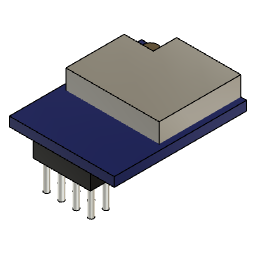
MLH3 v1.0 (Autodesk Fusion 360 archive; units mm, degrees)
design "RA-02"
Autodesk Fusion 360 part; units mm, degrees
sketch "Esquisse1" plane through (0, 0, 0) normal (0, 0, 1) x (1, 0, 0) in component "LoRa RA-02"
  line L0 (0, 0) -> (18, 0)
  line L1 (18, 0) -> (18, -22.7)
  line L2 (18, -22.7) -> (0, -22.7)
  line L3 (0, -22.7) -> (0, 0)
  line L4 (1, 0) -> (17, 0)
  line L5 (17, 0) -> (17, -14)
  line L6 (17, -14) -> (1, -14)
  line L7 (1, -14) -> (1, 0)
  line L8 (13.9, -22.7) -> (4.1, -22.7)
  line L9 (4.1, -22.7) -> (4.1, -17.7)
  line L10 (4.1, -17.7) -> (13.9, -17.7)
  line L11 (13.9, -17.7) -> (13.9, -22.7)
  line L12 (1, 0) -> (6, 0)
  line L13 (6, 0) -> (6, -4)
  line L14 (6, -4) -> (1, -4)
  line L15 (1, -4) -> (1, 0)
  circle A0 centre (3.5142, -2) radius 1.25
  circle A1 centre (5.2, -21.5) radius 0.445
  circle A2 centre (7.74, -21.5) radius 0.445
  circle A3 centre (10.28, -21.5) radius 0.445
  circle A4 centre (12.82, -21.5) radius 0.445
  circle A5 centre (5.2, -18.96) radius 0.445
  circle A6 centre (7.74, -18.96) radius 0.445
  circle A7 centre (10.28, -18.96) radius 0.445
  circle A8 centre (12.82, -18.96) radius 0.445
  dimension "d1" = 18
  dimension "d2" = 22.7
  dimension "d3" = 16
  dimension "d4" = 14
  dimension "d5" = 9.8
  dimension "d6" = 5
  dimension "d7" = 5
  dimension "d8" = 4
  dimension "d9" = 2.5
  dimension "d18" = 0.89
  dimension "d21" = 7.62
  dimension "d22" = 2.54
  dimension "d23" = 1.2
  dimension "d24" = 1.1
  constraint horizontal L0
  constraint vertical L1
  constraint horizontal L2
  constraint vertical L3
  constraint coincident L0.start L3.end
  constraint horizontal L4
  constraint vertical L5
  constraint horizontal L6
  constraint vertical L7
  constraint coincident L0 L4.start
  constraint midpoint L0 L4
  constraint horizontal L8
  constraint vertical L9
  constraint horizontal L10
  constraint vertical L11
  constraint coincident L2 L8.start
  constraint midpoint L2 L8
  constraint horizontal L12
  constraint vertical L13
  constraint horizontal L14
  constraint vertical L15
  measures "d1" distance of L0.start L0.end
  measures "d2" distance of L0.start L2.end
  measures "d3" distance of L4.start L4.end
  measures "d4" distance of L4.start L6.end
  measures "d5" distance of L8.start L8.end
  measures "d6" distance of L8.start L10.end
  measures "d7" distance of L4.start L12.end
  measures "d8" distance of L4.start L14.end
  measures "d9" diameter of A0
  measures "d18" diameter of A1
  measures "d23" distance of L2 A1.centre
  measures "d24" distance of L9 A1.centre
extrude "Extrusion1" add sketch "Esquisse1" along normal blind 1.6 contours L0 L1 L2 L3 L5 L6 L7 L9 L10 L11 L15 | L0 L4 L7 L12 L13 L14 L15 | L0 L4 L5 L6 L7 L13 L14 | L2 L8 L9 L10 L11 | A0 | A1 | A2 | A3 | A4 | A5 | A6 | A7 | A8 makes body 1 in component "LoRa RA-02"
extrude "Extrusion2" add sketch "Esquisse1" against normal blind 2.6 separate body contours L2 L8 L9 L10 L11 | A1 | A2 | A3 | A4 | A5 | A6 | A7 | A8 makes body 2 in component "LoRa RA-02"
extrude "Extrusion3" add sketch "Esquisse1" along normal blind 4.9 separate body contours L0 L4 L5 L6 L7 L13 L14 makes body 3 in component "LoRa RA-02"
extrude "Extrusion4" add sketch "Esquisse1" along normal blind 3 separate body contours A0 makes body 4 in component "LoRa RA-02"
extrude "Extrusion5" add sketch "Esquisse1" against normal blind 5 from surface at -2.6 separate body contours A1 | A2 | A3 | A4 | A5 | A6 | A7 | A8 makes body 5 at (10.077, -19.356, -4.2667) makes body 6 at (8.1712, -21.6098, -5.9333) makes body 7 at (12.617, -21.896, -4.2667) makes body 8 at (8.1712, -19.0698, -5.9333) makes body 9 at (12.617, -19.356, -4.2667) makes body 10 at (5.6312, -21.6098, -5.9333) makes body 11 at (10.077, -21.896, -4.2667) makes body 12 at (5.6312, -19.0698, -5.9333) in component "LoRa RA-02"
component "LoRa RA-02" placed x (1, 0, 0) y (0, 1, 0) z (0, 0, 1) at (0, 0, 0)
named bodies: "PCB", "connecteur", "SX11278", "IPX"

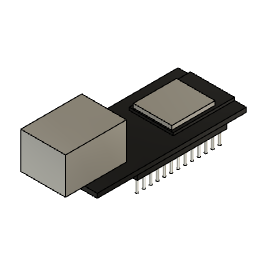
design "WT32-ETH01"
Autodesk Fusion 360 part; units mm, degrees
sketch "Esquisse1" plane through (0, 0, 0) normal (0, 0, 1) x (1, 0, 0) in component "WT32-ETH01"
  line L0 (-12.6, 31.1) -> (12.6, 31.1)
  line L1 (12.6, 31.1) -> (12.6, -23.9)
  line L2 (12.6, -23.9) -> (-12.6, -23.9)
  line L3 (-12.6, -23.9) -> (-12.6, 31.1)
  line L4 (12.6, -9.1479) -> (10.7452, -9.1479)
  line L5 (10.7452, -9.1479) -> (10.7452, 23.8669)
  line L6 (10.7452, 23.8669) -> (12.6, 23.8669)
  line L7 (12.6, 23.8669) -> (12.6, -9.1479)
  line L8 (-12.6, -9.1839) -> (-11, -9.1839)
  line L9 (-11, -9.1839) -> (-11, 24)
  line L10 (-11, 24) -> (-12.6, 24)
  line L11 (-12.6, 24) -> (-12.6, -9.1839)
  circle A0 centre (-11.55, -8) radius 0.445
  circle A1 centre (11.31, -8) radius 0.445
  circle A2 centre (-11.55, -5.46) radius 0.445
  circle A3 centre (11.31, -5.46) radius 0.445
  circle A4 centre (-11.55, -2.92) radius 0.445
  circle A5 centre (11.31, -2.92) radius 0.445
  circle A6 centre (-11.55, -0.38) radius 0.445
  circle A7 centre (11.31, -0.38) radius 0.445
  circle A8 centre (-11.55, 2.16) radius 0.445
  circle A9 centre (11.31, 2.16) radius 0.445
  circle A10 centre (-11.55, 4.7) radius 0.445
  circle A11 centre (11.31, 4.7) radius 0.445
  circle A12 centre (-11.55, 7.24) radius 0.445
  circle A13 centre (11.31, 7.24) radius 0.445
  circle A14 centre (-11.55, 9.78) radius 0.445
  circle A15 centre (11.31, 9.78) radius 0.445
  circle A16 centre (-11.55, 12.32) radius 0.445
  circle A17 centre (11.31, 12.32) radius 0.445
  circle A18 centre (-11.55, 14.86) radius 0.445
  circle A19 centre (11.31, 14.86) radius 0.445
  circle A20 centre (-11.55, 17.4) radius 0.445
  circle A21 centre (11.31, 17.4) radius 0.445
  circle A22 centre (-11.55, 19.94) radius 0.445
  circle A23 centre (11.31, 19.94) radius 0.445
  circle A24 centre (-11.55, 22.48) radius 0.445
  circle A25 centre (11.31, 22.48) radius 0.445
  dimension "d1" = 25.2
  dimension "d2" = 55
  dimension "d13" = 0.89
  dimension "d16" = 22.86
  dimension "d17" = 30.48
  dimension "d18" = 1.05
  constraint horizontal L0
  constraint vertical L1
  constraint horizontal L2
  constraint vertical L3
  constraint horizontal L4
  constraint vertical L5
  constraint horizontal L6
  constraint vertical L7
  constraint coincident L1 L4.start
  constraint horizontal L8
  constraint vertical L9
  constraint horizontal L10
  constraint vertical L11
  constraint coincident L3 L8.start
  measures "d1" distance of L0.start L0.end
  measures "d2" distance of L0.start L2.end
  measures "d13" diameter of A0
  measures "d18" distance of L11 A0.centre
extrude "Extrusion1" add sketch "Esquisse1" along normal blind 1.6 contours L0 L1 L2 L3 L4 L5 L6 L8 L9 L10 | L3 L8 L9 L10 L11 | L1 L4 L5 L6 L7 | A0 | A1 | A2 | A3 | A4 | A5 | A6 | A7 | A8 | A9 | A10 | A11 | A12 | A13 | A14 | A15 | A16 | A17 | A18 | A19 | A20 | A21 | A22 | A23 | A24 | A25 makes body 1 in component "WT32-ETH01"
extrude "Extrusion2" add sketch "Esquisse1" against normal blind 1.7 separate body contours L3 L8 L9 L10 L11 | L1 L4 L5 L6 L7 | A0 | A1 | A2 | A3 | A4 | A5 | A6 | A7 | A8 | A9 | A10 | A11 | A12 | A13 | A14 | A15 | A16 | A17 | A18 | A19 | A20 | A21 | A22 | A23 | A24 | A25 makes body 2 at (11.3634, 12.862, 0) makes body 3 at (-12.6, 1.8774, -0.5667) in component "WT32-ETH01"
sketch "Esquisse2" plane through (0, 0, 1.6) normal (0, 0, 1) x (-1, 0, 0) in component "WT32-ETH01"
  line L0 (12.6, -31.1) -> (12.6, 23.9)
  line L1 (12.6, 23.9) -> (-12.6, 23.9)
  line L2 (-12.6, 23.9) -> (-12.6, -31.1)
  line L3 (-12.6, -31.1) -> (12.6, -31.1)
  line L4 (8, -8.5) -> (-8.2548, -8.5)
  line L5 (-8.2548, -8.5) -> (-8.2548, -31.1)
  line L6 (-8.2548, -31.1) -> (8, -31.1)
  line L7 (8, -31.1) -> (8, -8.5)
  line L8 (8.5, 8.5) -> (-8, 8.5)
  line L9 (-8, 8.5) -> (-8, 31)
  line L10 (-8, 31) -> (8.5, 31)
  line L11 (8.5, 31) -> (8.5, 8.5)
  line L12 (7, -9) -> (-7.213, -9)
  line L13 (-7.213, -9) -> (-7.213, -24.9545)
  line L14 (-7.213, -24.9545) -> (7, -24.9545)
  line L15 (7, -24.9545) -> (7, -9)
  constraint horizontal L4
  constraint vertical L5
  constraint horizontal L6
  constraint vertical L7
  constraint coincident L3 L5.end
  constraint horizontal L8
  constraint vertical L9
  constraint horizontal L10
  constraint vertical L11
  constraint horizontal L12
  constraint vertical L13
  constraint horizontal L14
  constraint vertical L15
extrude "Extrusion3" add sketch "Esquisse2" along normal blind 13.5 separate body contours L1 L8 L9 L11 | L1 L9 L10 L11 makes body 4 in component "WT32-ETH01"
extrude "Extrusion4" add sketch "Esquisse2" along normal blind 1 separate body contours L3 L4 L5 L6 L7 makes body 5 in component "WT32-ETH01"
extrude "Extrusion5" add sketch "Esquisse2" along normal blind 2.5 separate body contours L12 L13 L14 L15 makes body 6 in component "WT32-ETH01"
extrude "Extrusion6" add sketch "Esquisse1" against normal blind 5 from surface at -1.7 separate body contours A0 | A1 | A2 | A3 | A4 | A5 | A6 | A7 | A8 | A9 | A10 | A11 | A12 | A13 | A14 | A15 | A16 | A17 | A18 | A19 | A20 | A21 | A22 | A23 | A24 | A25 makes body 7 at (-11.1056, -2.9422, -5.0333) makes body 8 at (-11.4295, 7.6684, -5.0333) makes body 9 at (-11.753, 17.004, -3.3667) makes body 10 at (11.107, 19.544, -3.3667) makes body 11 at (11.7412, 9.8898, -5.0333) makes body 12 at (11.4305, 0.0484, -5.0333) makes body 13 at (11.4305, -7.5716, -5.0333) makes body 14 at (11.7544, 2.1378, -5.0333) makes body 15 at (11.7412, 12.4298, -5.0333) makes body 16 at (11.107, 22.084, -3.3667) makes body 17 at (-11.1188, 14.9698, -5.0333) makes body 18 at (-11.4295, 5.1284, -5.0333) makes body 19 at (-11.4295, -7.5716, -5.0333) makes body 20 at (-11.4295, 0.0484, -5.0333) makes body 21 at (-11.1188, 9.8898, -5.0333) makes body 22 at (-11.753, 19.544, -3.3667) makes body 23 at (11.107, 17.004, -3.3667) makes body 24 at (11.4305, 7.6684, -5.0333) makes body 25 at (11.7544, -2.9422, -5.0333) makes body 26 at (11.4305, -5.0316, -5.0333) makes body 27 at (11.4305, 5.1284, -5.0333) makes body 28 at (11.7412, 14.9698, -5.0333) makes body 29 at (-11.753, 22.084, -3.3667) makes body 30 at (-11.1188, 12.4298, -5.0333) makes body 31 at (-11.1056, 2.1378, -5.0333) makes body 32 at (-11.4295, -5.0316, -5.0333) in component "WT32-ETH01"
component "WT32-ETH01" placed x (1, 0, 0) y (0, 1, 0) z (0, 0, 1) at (0, 0, 0)
named bodies: "PCB", "J1", "J2", "RJ45", "Antenna", "ESP32-wroom"
